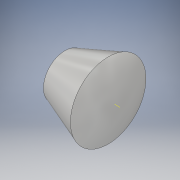
# Autodesk Inventor part: capcule
Saved by Autodesk Inventor 2019.1 (Build 231200000, 200)
## iProperties
Created: 2018-12-21
Part Number: capcule
Material: 鋼、炭素鋼
Document SubType Name: Modeling
Designer: Masaya
Density: 7.85 g/cm^3
Appearance: 機械加工 - アルミニウム
Author: Masaya
Autodesk Inventor part; units mm, degrees
ref_plane "YZ Plane" through (0, 0, 0) normal (1, 0, 0) x (0, 1, 0)
ref_plane "XZ Plane" through (0, 0, 0) normal (0, 1, 0) x (-1, 0, 0)
ref_plane "XY Plane" through (0, 0, 0) normal (0, 0, 1) x (1, 0, 0)
sketch "スケッチ1" plane through (0, 0, 0) normal (0, 1, 0) x (-1, 0, 0)
  line L0 (0, 200) -> (-400, 350)
  line L1 (0, 200) -> (0, 0)
  arc A0 (-400, 350) -> (-463.2503, 0) centre (536.7497, 0) ccw
  line L2 (739.8868, 0) -> (-682.0729, 0) projected
  dimension "d0" = 350
  dimension "d1" = 200
  dimension "d2" = 400
  dimension "d3" = 1000
  constraints: 4 end point, 2 point on circle, 2 point on line, 1 centre point, 1 vertical
  measures "d0" vertical distance of L1.end L0.end
  measures "d1" distance of L1.end L0.start
  measures "d2" distance from line of L0.end L1
  measures "d3" radius of A0
revolve "回転1" add sketch "スケッチ1" angle 360 about axis through (-10, 0, 0) along (1, 0, 0)
